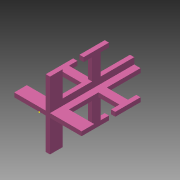
# Autodesk Inventor part: Pièce3
Saved by Autodesk Inventor 2015 (Build 190159000, 159)
## iProperties
Created: 2019-02-09
Part Number: Pièce3
Material: Générique
Document SubType Name: Modeling
Designer: Naly jérémie
Density: 1 g/cm^3
Appearance: Rose
Author: Naly jérémie
Autodesk Inventor part; units mm, degrees
ref_plane "YZ Plane" through (0, 0, 0) normal (1, 0, 0) x (0, 1, 0)
ref_plane "XZ Plane" through (0, 0, 0) normal (0, 1, 0) x (-1, 0, 0)
ref_plane "XY Plane" through (0, 0, 0) normal (0, 0, 1) x (1, 0, 0)
sketch "Esquisse1" plane through (0, 0, 0) normal (0, 0, 1) x (1, 0, 0)
  point P0 (0, 0)
sketch "Esquisse2" plane through (0, 0, 0) normal (0, 0, 1) x (1, 0, 0)
  line L0 (0, 0) -> (20, 0)
  line L1 (20, 0) -> (20, 100)
  line L2 (20, 100) -> (0, 100)
  line L3 (0, 100) -> (0, 0)
  dimension "d0" = 100
  dimension "d1" = 20
  constraints: 8 end point, 2 parallel, 1 horizontal, 1 perpendicular
  measures "d0" distance of L2.end L0.start
  measures "d1" distance of L1.end L2.end
extrude "Extrusion1" add sketch "Esquisse2" along normal blind 5
sketch "Esquisse3" plane through (0, 0, 5) normal (0, 0, 1) x (1, 0, 0)
  line L0 (20, 100) -> (0, 100) projected
  line L1 (0, 0) -> (20, 0) projected
  line L2 (7.5, 100) -> (12.5, 100)
  line L3 (12.5, 100) -> (12.5, 0)
  line L4 (12.5, 0) -> (7.5, 0)
  line L5 (7.5, 0) -> (7.5, 100)
  line L6 (20, 0) -> (20, 100) projected
  line L7 (0, 100) -> (0, 0) projected
  dimension "d4" = 7.5
  dimension "d5" = 7.5
  constraints: 8 end point, 2 parallel, 2 point on line, 1 horizontal, 1 perpendicular
  measures "d4" distance between parallel lines of L6 L3
  measures "d5" distance between parallel lines of L7 L5
extrude "Extrusion2" add sketch "Esquisse3" along normal blind 7.5 and the other way blind 12.5 contours L3 L1 L5 L0
sketch "Esquisse4" plane through (0, 0, 12.5) normal (0, 0, 1) x (1, 0, 0)
  line L0 (12.5, 0) -> (12.5, 100) projected
  line L1 (7.5, 0) -> (12.5, 0)
  line L2 (12.5, 0) -> (12.5, 15)
  line L3 (12.5, 15) -> (7.5, 15)
  line L4 (7.5, 15) -> (7.5, 0)
  point P0 (0, 0)
  dimension "d10" = 15
  constraints: 8 end point, 2 parallel, 1 horizontal, 1 perpendicular, 1 point on line
  measures "d10" distance between parallel lines of L1 L3
extrude "Extrusion3" add sketch "Esquisse4" along normal blind 30 and the other way blind 50
sketch "Esquisse5" plane through (0, 0, 0) normal (-1, 0, 0) x (0, 0, 1)
  line L0 (5, 100) -> (5, 0) projected
  line L1 (0, 0) -> (5, 0)
  line L2 (5, 0) -> (5, 15)
  line L3 (5, 15) -> (0, 15)
  line L4 (0, 15) -> (0, 0)
  dimension "d15" = 15
  constraints: 8 end point, 2 parallel, 1 horizontal, 1 perpendicular, 1 point on line
  measures "d15" distance between parallel lines of L1 L3
extrude "Extrusion4" add sketch "Esquisse5" along normal blind 30 and the other way blind 50
sketch "Esquisse6" plane through (0, 100, 0) normal (-1, 0, 0) x (0, 0, 1)
  line L0 (5, 0) -> (5, -85) projected
  line L1 (0, -50) -> (5, -50)
  line L2 (5, -50) -> (5, -40)
  line L3 (5, -40) -> (0, -40)
  line L4 (0, -40) -> (0, -50)
  line L5 (0, 0) -> (5, 0) projected
  line L6 (0, -85) -> (5, -85) projected
  point P0 (0, -100)
  dimension "d20" = 40
  dimension "d22" = 35
  constraints: 8 end point, 2 parallel, 1 horizontal, 1 perpendicular, 1 point on line
  measures "d20" distance between parallel lines of L5 L3
  measures "d22" distance between parallel lines of L6 L1
extrude "Extrusion5" add sketch "Esquisse6" along normal blind 30 and the other way blind 50
sketch "Esquisse7" plane through (20, 60, 5) normal (0, 1, 0) x (1, 0, 0)
  line L0 (-20, 5) -> (-50, 5) projected
  line L1 (-50, 0) -> (-45, 0)
  line L2 (-45, 0) -> (-45, 5)
  line L3 (-45, 5) -> (-50, 5)
  line L4 (-50, 5) -> (-50, 0)
  dimension "d27" = 5
  dimension "d28" = 5
  dimension "d29" = 5
  constraints: 8 end point, 2 parallel, 1 horizontal, 1 perpendicular, 1 point on line
  measures "d27" distance of L1.end L2.end
  measures "d28" distance between parallel lines of L0 L1
  measures "d29" distance between parallel lines of L4 L2
extrude "Extrusion6" add sketch "Esquisse7" along normal blind 10 and the other way blind 20
sketch "Esquisse8" plane through (20, 60, 5) normal (0, 1, 0) x (1, 0, 0)
  line L0 (30, 0) -> (25, 0)
  line L1 (25, 0) -> (25, 5)
  line L2 (25, 5) -> (30, 5)
  line L3 (30, 5) -> (30, 0)
  point P0 (-20, 5)
  dimension "d34" = 5
  dimension "d35" = 5
  constraints: 8 end point, 2 parallel, 1 horizontal, 1 perpendicular
  measures "d34" distance between parallel lines of L3 L1
  measures "d35" distance between parallel lines of L2 L0
extrude "Extrusion7" add sketch "Esquisse8" along normal blind 10 and the other way blind 20
sketch "Esquisse9" plane through (0, 0, -7.5) normal (0, 0, -1) x (-1, 0, 0)
  line L0 (-7.5, 15) -> (-7.5, 100) projected
  line L1 (-12.5, 60) -> (-7.5, 60)
  line L2 (-7.5, 60) -> (-7.5, 50)
  line L3 (-7.5, 50) -> (-12.5, 50)
  line L4 (-12.5, 50) -> (-12.5, 60)
  line L5 (-7.5, 100) -> (-12.5, 100) projected
  line L6 (-12.5, 15) -> (-7.5, 15) projected
  point P0 (0, 0)
  dimension "d40" = 5
  dimension "d41" = 40
  dimension "d42" = 35
  constraints: 8 end point, 2 parallel, 1 horizontal, 1 perpendicular, 1 point on line
  measures "d40" distance between parallel lines of L4 L2
  measures "d41" distance between parallel lines of L5 L1
  measures "d42" distance between parallel lines of L6 L3
extrude "Extrusion8" add sketch "Esquisse9" along normal blind 30 and the other way blind 50
sketch "Esquisse10" plane through (7.5, 60, 12.5) normal (0, 1, 0) x (1, 0, 0)
  line L0 (0, 0) -> (0, -30) projected
  line L1 (5, -30) -> (0, -30)
  line L2 (0, -30) -> (0, -25)
  line L3 (0, -25) -> (5, -25)
  line L4 (5, -25) -> (5, -30)
  point P0 (-7.5, 12.5)
  dimension "d47" = 5
  constraints: 8 end point, 2 parallel, 1 horizontal, 1 perpendicular, 1 point on line
  measures "d47" distance between parallel lines of L1 L3
extrude "Extrusion9" add sketch "Esquisse10" along normal blind 10 and the other way blind 20
sketch "Esquisse11" plane through (7.5, 60, -7.5) normal (0, 1, 0) x (1, 0, 0)
  line L0 (5, 0) -> (5, 30) projected
  line L1 (0, 30) -> (5, 30)
  line L2 (5, 30) -> (5, 25)
  line L3 (5, 25) -> (0, 25)
  line L4 (0, 25) -> (0, 30)
  point P0 (-7.5, -7.5)
  dimension "d52" = 5
  constraints: 8 end point, 2 parallel, 1 horizontal, 1 perpendicular, 1 point on line
  measures "d52" distance between parallel lines of L1 L3
extrude "Extrusion10" add sketch "Esquisse11" along normal blind 10 and the other way blind 20
